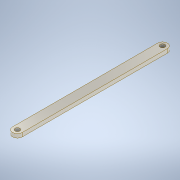
# Autodesk Inventor part: pod
Saved by Autodesk Inventor 2022 (Build 260153000, 153)
## iProperties
Created: 2022-06-18
Part Number: pod
Material: Titanio
Document SubType Name: Modeling
Designer: corra
Mass: 18.04 g
Surface Area: 28.8 cm^2
Volume: 4 cm^3
Density: 4.51 g/cm^3
Appearance: Titanio
Author: corra
Autodesk Inventor part; units mm, degrees
ref_plane "YZ Plane" through (0, 0, 0) normal (1, 0, 0) x (0, 1, 0)
ref_plane "XZ Plane" through (0, 0, 0) normal (0, 1, 0) x (-1, 0, 0)
ref_plane "XY Plane" through (0, 0, 0) normal (0, 0, 1) x (1, 0, 0)
sketch "Schizzo1" plane through (0, 0, 0) normal (0, 1, 0) x (-1, 0, 0)
  line L0 (0, 0) -> (10, 0)
  line L1 (10, 0) -> (10, -150)
  line L2 (10, -150) -> (0, -150)
  line L3 (0, -150) -> (0, 0)
  dimension "d0" = 150
  dimension "d1" = 10
  constraints: 8 end point, 2 parallel, 1 horizontal, 1 perpendicular
  measures "d0" distance of L0.end L1.end
  measures "d1" distance of L1.end L2.end
extrude "Estrusione1" add sketch "Schizzo1" along normal blind 4
sketch "Schizzo2" plane through (0, 4, 0) normal (0, 1, 0) x (1, 0, 0)
  line L0 (-10, 0) -> (0, 0) projected
  circle A0 centre (-5, 0) radius 5
  circle A1 centre (-5, 0) radius 2.5
  line L1 (0, 150) -> (-10, 150) projected
  circle A2 centre (-5, 150) radius 5
  circle A3 centre (-5, 150) radius 2.5
  point P0 (-7.5, 150)
  point P1 (-2.5, 150)
  point P2 (-2.5, 0)
  point P3 (-7.5, 0)
  dimension "d4" = 5
  dimension "d5" = 5
  constraints: 2 centre point, 2 coincident, 2 horizontal alignment, 2 midpoint, 4 other
  measures "d4" diameter of A1
  measures "d5" diameter of A3
extrude "Estrusione2" add sketch "Schizzo2" against normal up to surface (4 mm away) contours A1 L0 A0 | L0 A0 A1 | A2 L1 A3 | L1 A3 A2
extrude "Estrusione3" cut sketch "Schizzo2" against normal blind 10 contours L0 A1 | A3 L1 picked at (-4.3762, 0.5526) picked at (-4.7045, 148.822)
